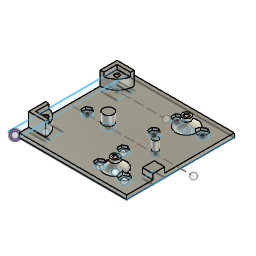
PlatinenhalterNEU v6 (Autodesk Fusion 360 design; units mm, degrees)
Autodesk Fusion 360 part; units mm, degrees
sketch "Skizze1" plane through (0, 0, 0) normal (0, 0, 1) x (1, 0, 0)
  line L0 (0, 0) -> (85, 0)
  line L1 (85, 0) -> (85, 82)
  line L2 (85, 82) -> (0, 82)
  line L3 (53, 82) -> (53, 0) construction
  line L4 (3, 41) -> (95, 41) construction
  circle A0 centre (53, 70.5) radius 1.75
  circle A1 centre (53, 52.7) radius 1.75
  circle A2 centre (71.9985, 70.7359) radius 1.75
  line L5 (53, 56.1641) -> (50, 54.4321)
  line L6 (50, 54.4321) -> (50, 50.9679)
  line L7 (50, 50.9679) -> (53, 49.2359)
  line L8 (53, 49.2359) -> (56, 50.9679)
  line L9 (56, 50.9679) -> (56, 54.4321)
  line L10 (56, 54.4321) -> (53, 56.1641)
  line L11 (50, 72.2321) -> (50, 68.7679)
  line L12 (50, 68.7679) -> (53, 67.0359)
  line L13 (53, 67.0359) -> (56, 68.7679)
  line L14 (56, 68.7679) -> (56, 72.2321)
  line L15 (56, 72.2321) -> (53, 73.9641)
  line L16 (53, 73.9641) -> (50, 72.2321)
  line L17 (75.4985, 72.7566) -> (71.9985, 74.7773)
  line L18 (71.9985, 74.7773) -> (68.4985, 72.7566)
  line L19 (68.4985, 72.7566) -> (68.4985, 68.7152)
  line L20 (68.4985, 68.7152) -> (71.9985, 66.6944)
  line L21 (71.9985, 66.6944) -> (75.4985, 68.7152)
  line L22 (75.4985, 68.7152) -> (75.4985, 72.7566)
  line L23 (56, 27.5679) -> (53, 25.8359)
  line L24 (53, 25.8359) -> (50, 27.5679)
  line L25 (50, 27.5679) -> (50, 31.0321)
  line L26 (50, 31.0321) -> (53, 32.7641)
  line L27 (56, 31.0321) -> (56, 27.5679)
  line L28 (53, 32.7641) -> (56, 31.0321)
  circle A3 centre (53, 29.3) radius 1.75
  line L29 (56, 9.7679) -> (53, 8.0359)
  line L30 (53, 8.0359) -> (50, 9.7679)
  line L31 (50, 9.7679) -> (50, 13.2321)
  line L32 (50, 13.2321) -> (53, 14.9641)
  line L33 (56, 13.2321) -> (56, 9.7679)
  line L34 (53, 14.9641) -> (56, 13.2321)
  circle A4 centre (53, 11.5) radius 1.75
  line L35 (75.4985, 13.2848) -> (75.4985, 9.2434)
  line L36 (75.4985, 9.2434) -> (71.9985, 7.2227)
  line L37 (71.9985, 7.2227) -> (68.4985, 9.2434)
  line L38 (68.4985, 9.2434) -> (68.4985, 13.2848)
  line L39 (71.9985, 15.3056) -> (75.4985, 13.2848)
  line L40 (68.4985, 13.2848) -> (71.9985, 15.3056)
  circle A5 centre (71.9985, 11.2641) radius 1.75
  line L41 (3, 7.3) -> (16, 7.3)
  line L42 (16, 7.3) -> (16, 20.3)
  line L43 (16, 20.3) -> (3, 20.3)
  line L44 (3, 20.3) -> (3, 7.3)
  line L45 (3, 74.7) -> (16, 74.7)
  line L46 (16, 74.7) -> (16, 61.7)
  line L47 (16, 61.7) -> (3, 61.7)
  line L48 (3, 61.7) -> (3, 74.7)
  line L49 (16, 72) -> (5.7, 72)
  line L50 (5.7, 72) -> (5.7, 61.7)
  line L51 (16, 10) -> (5.7, 10)
  line L52 (5.7, 20.3) -> (5.7, 10)
  circle A6 centre (14, 41) radius 1.75
  line L53 (14, 44.4641) -> (11, 42.7321)
  line L54 (11, 42.7321) -> (11, 39.2679)
  line L55 (11, 39.2679) -> (14, 37.5359)
  line L56 (14, 37.5359) -> (17, 39.2679)
  line L57 (17, 39.2679) -> (17, 42.7321)
  line L58 (17, 42.7321) -> (14, 44.4641)
  line L59 (9.5, 74.7) -> (9.5, 61.7) construction
  circle A7 centre (9.5, 68.2) radius 1.4
  circle A8 centre (9.5, 13.8) radius 1.4
  line L60 (3, 68.2) -> (47, 68.2) construction
  circle A9 centre (62.5, 68.2) radius 1.4
  circle A10 centre (62.5, 68.2) radius 3.25
  circle A11 centre (62.5, 13.8) radius 3.25
  circle A12 centre (62.5, 13.8) radius 1.4
  circle A13 centre (66, 41) radius 2.25
  circle A14 centre (30, 41) radius 4
  line L61 (85, 29) -> (77, 29)
  line L62 (77, 29) -> (77, 20)
  line L63 (77, 20) -> (85, 20)
  line L64 (85, 20) -> (85, 29)
  line L65 (0, 82) -> (-5, 82)
  line L66 (-5, 82) -> (-5, 0)
  line L67 (-5, 0) -> (0, 0)
  line L68 (3, 7.3) -> (3, 20.3)
  line L69 (3, 61.7) -> (3, 74.7)
  line L70 (3, 74.7) -> (3, 61.7)
  line L71 (3, 20.3) -> (3, 7.3)
  line L72 (5.7, 72) -> (16, 72)
  line L73 (5.7, 10) -> (16, 10)
  line L74 (3, 74.7) -> (3, 82)
  line L75 (3, 61.7) -> (3, 20.3)
  line L76 (3, 7.3) -> (3, 0)
  point P0 (53, 52.7)
  point P1 (53, 70.5)
  point P2 (71.9985, 70.7359)
  point P3 (14, 41)
  dimension "d2" = 82
  dimension "d4" = 3.5
  dimension "d5" = 3.5
  dimension "d6" = 11.5
  dimension "d7" = 17.8
  dimension "d8" = 3.5
  dimension "d9" = 19
  dimension "d10" = 3
  dimension "d11" = 3
  dimension "d12" = 3.5
  dimension "d17" = 31
  dimension "d18" = 31
  dimension "d21" = 13
  dimension "d22" = 13
  dimension "d23" = 13
  dimension "d24" = 13
  dimension "d25" = 2.7
  dimension "d26" = 2.7
  dimension "d27" = 2.7
  dimension "d28" = 2.7
  dimension "d29" = 3.5
  dimension "d31" = 39
  dimension "d32" = 3
  dimension "d33" = 2.8
  dimension "d34" = 2.8
  dimension "d35" = 53
  dimension "d36" = 6.5
  dimension "d44" = 4.5
  dimension "d45" = 8
  dimension "d46" = 27
  dimension "d47" = 19
  dimension "d48" = 9
  dimension "d49" = 8
  dimension "d54" = 37
  dimension "d58" = 82
  dimension "d59" = 19
  dimension "d60" = 32
  dimension "d61" = 13.8
  constraint horizontal L0
  constraint vertical L1
  constraint horizontal L2
  constraint vertical L70
  constraint coincident L0.start L67.end
  constraint coincident L2 L3.start
  constraint coincident L0 L3.end
  constraint perpendicular L0 L3
  constraint perpendicular L4 L70
  constraint coincident L3 P1
  constraint coincident L3 P0
  constraint coincident P0 A1.centre
  constraint coincident P1 A0.centre
  constraint coincident P2 A2.centre
  constraint parallel L3 L9
  constraint parallel L3 L14
  constraint parallel L3 L19
  constraint symmetric L4 A0 A4
  constraint symmetric L4 A1 A3
  constraint symmetric L4 A2 A5
  constraint symmetric L4 L5.start L23.end
  constraint symmetric L4 L5.end L24.end
  constraint symmetric L4 L6.end L25.end
  constraint symmetric L4 L7.end L26.end
  constraint symmetric L4 L8.end L27.start
  constraint symmetric L4 L9.end L23.start
  constraint symmetric L4 L11.start L30.end
  constraint symmetric L4 L11.end L31.end
  constraint symmetric L4 L12.end L32.end
  constraint symmetric L4 L13.end L33.start
  constraint symmetric L4 L14.end L29.start
  constraint symmetric L4 L15.end L29.end
  constraint symmetric L4 L17.start L35.end
  constraint symmetric L4 L17.end L36.end
  constraint symmetric L4 L18.end L37.end
  constraint symmetric L4 L19.end L38.end
  constraint symmetric L4 L20.end L39.start
  constraint symmetric L4 L21.end L35.start
  constraint perpendicular L1 L73
  constraint perpendicular L1 L72
  constraint horizontal L41
  constraint vertical L42
  constraint horizontal L43
  constraint vertical L44
  constraint coincident L41.start L70
  constraint horizontal L45
  constraint vertical L46
  constraint horizontal L47
  constraint vertical L48
  constraint coincident L46 L49.start
  constraint coincident L47 L50.end
  constraint perpendicular L47 L50
  constraint coincident L42 L51.start
  constraint coincident L43 L52.start
  constraint perpendicular L41 L52
  constraint coincident L4 P3
  constraint coincident P3 A6.centre
  constraint parallel L3 L57
  constraint midpoint L45 L59.start
  constraint midpoint L47 L59.end
  constraint midpoint L59 A7.centre
  constraint symmetric L4 A7 A8
  constraint midpoint L48 L60.start
  constraint perpendicular L48 L60
  constraint coincident L60 A9.centre
  constraint concentric A9 A10
  constraint symmetric L4 A9 A12
  constraint symmetric L4 A10 A11
  constraint coincident L4 A13.centre
  constraint coincident L4 A14.centre
  constraint horizontal L61
  constraint vertical L62
  constraint horizontal L63
  constraint vertical L64
  constraint coincident L1 L61.start
  constraint horizontal L65
  constraint vertical L66
  constraint horizontal L67
  constraint vertical L68
  constraint collinear L68 L69
  constraint collinear L70 L71
  constraint coincident L4.start L70
  constraint coincident L2 L74.end
  constraint perpendicular L2 L74
  constraint coincident L0 L76.end
  constraint perpendicular L0 L76
  measures "d2" distance of L0.start L2.end
  measures "d4" diameter of A0
  measures "d5" diameter of A1
  measures "d6" distance of L2 P1
  measures "d7" distance of P1 P0
  measures "d8" diameter of A2
  measures "d9" distance of P1 P2
  measures "d10" distance of P0 L10
  measures "d11" distance of P1 L16
  measures "d12" distance of P2 L22
  measures "d17" distance of L4 L72
  measures "d18" distance of L4 L73
  measures "d21" distance of L41.start L41.end
  measures "d22" distance of L41.start L43.end
  measures "d23" distance of L45.start L45.end
  measures "d24" distance of L45.start L47.end
  measures "d25" distance of L41 L51
  measures "d26" distance of L52 L70
  measures "d27" distance of L50 L70
  measures "d28" distance of L45 L49
  measures "d29" diameter of A6
  measures "d31" distance of L3 P3
  measures "d32" distance of P3 L58
  measures "d33" diameter of A7
  measures "d34" diameter of A9
  measures "d35" distance of A7.centre A9.centre
  measures "d36" diameter of A10
  measures "d44" diameter of A13
  measures "d45" diameter of A14
  measures "d46" distance of A14.centre L70
  measures "d47" distance of L61 L73
  measures "d48" distance of L61 L63
  measures "d49" distance of L1 L62
  measures "d54" distance of L3 L46
  measures "d58" distance of L1 L76
  measures "d59" distance of L1 A13.centre
  measures "d60" distance of L1 L3
  measures "d61" distance of L2 A9.centre
extrude "Extrusion1" add sketch "Skizze1" along normal blind 3 contours L0 L1 L2 L41 L42 L43 L45 L46 L47 L61 L62 L63 L74 L75 L76 | L41 L42 L43 L44 L51 L52 L68 L71 L73 | L1 L61 L62 L63 L64 | L42 L43 L51 L52 L73 | L45 L46 L47 L48 L49 L50 L69 L70 L72 | L46 L47 L49 L50 L72 | A10 | A11 | A13 | A14
extrude "Extrusion2" add sketch "Skizze1" along normal blind 1 contours L5 L6 L7 L8 L9 L10 | L11 L12 L13 L14 L15 L16 | L17 L18 L19 L20 L21 L22 | L23 L24 L25 L26 L27 L28 | L29 L30 L31 L32 L33 L34 | L35 L36 L37 L38 L39 L40 | L53 L54 L55 L56 L57 L58
extrude "Extrusion3" add sketch "Skizze1" along normal blind 13.5 contours L41 L42 L43 L44 L51 L52 L68 L71 L73 | L45 L46 L47 L48 L49 L50 L69 L70 L72
extrude "Extrusion4" add sketch "Skizze1" along normal blind 10.3 contours L42 L43 L51 L52 L73 | L46 L47 L49 L50 L72 | A10 | A11 | A13 | A14
fillet "Abrundung1" radius 13 2 edges at (16, 61.7, 6.65) (16, 20.3, 6.65)
chamfer "Fase1" distance 0.5 angle 45 4 edges at (8.1947, 68.7063, 10.3) (8.1947, 14.3063, 10.3) (61.1947, 14.3063, 10.3) (61.1947, 68.7063, 10.3)
extrude "Extrusion5" add sketch "Skizze1" along normal blind 7.1 contours L1 L61 L62 L63 L64
fillet "Abrundung2" radius 5 tangency weight 0.5 2 edges at (59.4699, 14.9753, 3) (59.4699, 69.3753, 3)
